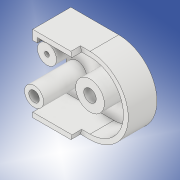
# Autodesk Inventor part: FA004
Saved by Autodesk Inventor 2017 SP1 (Build 210196100, 196)
## iProperties
Created: 2017-06-16
Part Number: FA004
Material: ABS Plastic
Document SubType Name: Modeling
Designer: Zach
Density: 1.06 g/cm^3
Appearance: CR White
Author: Zach
Autodesk Inventor part; units mm, degrees
ref_plane "YZ Plane" through (0, 0, 0) normal (1, 0, 0) x (0, 1, 0)
ref_plane "XZ Plane" through (0, 0, 0) normal (0, 1, 0) x (-1, 0, 0)
ref_plane "XY Plane" through (0, 0, 0) normal (0, 0, 1) x (1, 0, 0)
sketch "Sketch1" plane through (0, 0, 0) normal (0, 0, 1) x (1, 0, 0)
  line L0 (0, 0) -> (50, 0)
  line L1 (50, 0) -> (50, 80) construction
  line L2 (50, 80) -> (0, 80)
  line L3 (0, 80) -> (0, 0)
  circle A0 centre (50, 40) radius 40 construction
  arc A1 (50, 0) -> (50, 80) centre (50, 40) ccw
  dimension "d0" = 50
  dimension "d1" = 80
  dimension "d2" = 80
  constraints: 8 end point, 2 centre point, 2 parallel, 2 point on circle, 2 tangent, 1 horizontal, 1 midpoint, 1 perpendicular
  measures "d0" distance of L2.end L1.end
  measures "d1" distance of L1.end L0.end
  measures "d2" diameter of A0
extrude "Extrusion1" add sketch "Sketch1" along normal blind 40
sketch "Sketch2" plane through (0, 0, 40) normal (0, 0, 1) x (1, 0, 0)
  line L0 (50, 80) -> (0, 80) projected
  arc A0 (50, 0) -> (50, 80) centre (50, 40) ccw projected
  line L1 (0, 0) -> (50, 0) projected
  line L2 (0, 75) -> (50, 75)
  arc A1 (50, 5) -> (50, 75) centre (50, 40) ccw
  line L3 (50, 5) -> (0, 5)
  line L4 (0, 75) -> (0, 5)
  line L5 (0, 80) -> (0, 0) projected
  dimension "d5" = 5
  constraints: 6 end point, 2 point on circle, 1 centre point, 1 collinear, 2 other
  measures "d5" distance between parallel lines of L0 L2
extrude "Extrusion2" cut sketch "Sketch2" against normal blind 35 contours L2 A1 L3 L4
sketch "Sketch3" plane through (0, 0, 0) normal (-1, 0, 0) x (0, 0, 1)
  line L0 (0, 80) -> (0, 0) projected
  line L1 (40, 75) -> (40, 5) projected
  line L2 (0, 80) -> (40, 80)
  line L3 (40, 80) -> (40, 70)
  line L4 (40, 70) -> (0, 70)
  line L5 (0, 70) -> (0, 80)
  line L6 (0, 80) -> (10, 80)
  line L7 (10, 80) -> (10, 50)
  line L8 (10, 50) -> (0, 50)
  line L9 (0, 50) -> (0, 80)
  line L10 (0, 0) -> (40, 0) projected
  dimension "d8" = 10
  dimension "d9" = 10
  dimension "d10" = 50
  constraints: 16 end point, 4 parallel, 2 horizontal, 2 perpendicular, 1 point on line
  measures "d8" distance of L2.end L3.end
  measures "d9" distance of L7.end L8.end
  measures "d10" distance between parallel lines of L10 L8
extrude "Extrusion3" add sketch "Sketch3" against normal blind 5
sketch "Sketch4" plane through (0, 0, 40) normal (0, 0, 1) x (1, 0, 0)
  line L0 (50, 80) -> (50, 0)
  arc A0 (50, 0) -> (50, 80) centre (50, 40) ccw projected
  arc A1 (50, 0) -> (50, 80) centre (50, 40) ccw projected
  arc A2 (50, 0) -> (50, 80) centre (50, 40) ccw
  line L1 (50, 40) -> (40, 80)
  line L2 (50, 80) -> (0, 80) projected
  line L3 (40, 80) -> (50, 80)
  line L4 (50, 40) -> (40, 0)
  line L5 (0, 0) -> (50, 0) projected
  line L6 (40, 0) -> (50, 0)
  dimension "d15" = 10
  constraints: 10 end point, 2 collinear, 2 point on circle, 2 point on line, 1 centre point, 1 vertical, 1 vertical alignment
  measures "d15" distance of L0.start L1.end
extrude "Extrusion4" cut sketch "Sketch4" against normal blind 10
sketch "Sketch5" plane through (0, 0, 5) normal (0, 0, 1) x (1, 0, 0)
  circle A0 centre (11.5, 30) radius 10
  circle A1 centre (11.5, 30) radius 5.5
  line L0 (0, 0) -> (40, 0) projected
  line L1 (0, 5) -> (0, 50) projected
  dimension "d16" = 20
  dimension "d17" = 11
  dimension "d18" = 30
  dimension "d19" = 11.5
  constraints: 2 centre point, 1 coincident
  measures "d16" diameter of A0
  measures "d17" diameter of A1
  measures "d18" distance from line of L0 A0.centre
  measures "d19" distance from line of L1 A0.centre
extrude "Extrusion5" add sketch "Sketch5" along normal blind 45
sketch "Sketch6" plane through (0, 0, 5) normal (0, 0, 1) x (1, 0, 0)
  circle A0 centre (50, 40) radius 15
  circle A1 centre (50, 40) radius 6.5
  line L0 (0, 5) -> (0, 50) projected
  line L1 (0, 0) -> (40, 0) projected
  dimension "d22" = 30
  dimension "d23" = 13
  dimension "d24" = 50
  dimension "d25" = 40
  constraints: 2 centre point, 1 coincident
  measures "d22" diameter of A0
  measures "d23" diameter of A1
  measures "d24" distance from line of L0 A0.centre
  measures "d25" distance from line of L1 A0.centre
extrude "Extrusion6" add sketch "Sketch6" along normal blind 25
sketch "Sketch7" plane through (0, 0, 5) normal (0, 0, 1) x (1, 0, 0)
  circle A0 centre (15, 65) radius 10
  circle A1 centre (15, 65) radius 2.5
  line L0 (5, 75) -> (41.25, 75) projected
  line L1 (5, 70) -> (5, 50) projected
  point P0 (0, 0)
  dimension "d28" = 20
  dimension "d29" = 5
  constraints: 2 centre point, 2 tangent, 1 coincident
  measures "d28" diameter of A0
  measures "d29" diameter of A1
extrude "Extrusion7" add sketch "Sketch7" along normal blind 35
sketch "Sketch9" plane through (0, 0, 0) normal (0, 0, -1) x (-1, 0, 0)
  arc A0 (-15, 75) -> (-5, 65) centre (-15, 65) ccw projected
  arc A1 (-5, 65) -> (-15, 75) centre (-15, 65) ccw projected
  circle A2 centre (-15, 65) radius 2.5 projected
  circle A3 centre (-15, 65) radius 2.5 projected
  circle A4 centre (-15, 65) radius 7.5
  point P0 (0, 0)
  dimension "d34" = 15
  constraints: 1 centre point, 1 coincident
  measures "d34" diameter of A4
extrude "Extrusion9" cut sketch "Sketch9" against normal blind 30 contours A2 | A4
body "Solid1"
